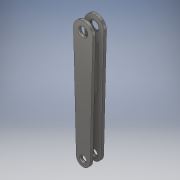
# Autodesk Inventor part: Upper Rocker Arm Spider Crab
Saved by Autodesk Inventor 2019 (Build 230136000, 136)
## iProperties
Created: 2019-08-25
Part Number: Upper Rocker Arm Spider Crab
Material: Steel, Mild
Document SubType Name: Modeling
Designer: DIBYOJYOTI
Density: 7.85 g/cm^3
Appearance: Semi-Polished
Mass: 46.5532 g
Surface Area: 51.0347 cm^2
Volume: 5.93034 cm^3
Author: DIBYOJYOTI
Autodesk Inventor part; units mm, degrees
ref_plane "YZ Plane" through (0, 0, 0) normal (1, 0, 0) x (0, 1, 0)
ref_plane "XZ Plane" through (0, 0, 0) normal (0, 1, 0) x (-1, 0, 0)
ref_plane "XY Plane" through (0, 0, 0) normal (0, 0, 1) x (1, 0, 0)
sketch "Sketch1" plane through (0, 0, 0) normal (0, 0, 1) x (1, 0, 0)
  circle A0 centre (0, 0) radius 2.05
  circle A1 centre (0, 80) radius 3.05
  arc A2 (6.9978, 79.8249) -> (-6.9978, 79.8249) centre (0, 80) ccw
  arc A3 (-5, 0) -> (5, 0) centre (0, 0) ccw
  line L0 (-5, 0) -> (-6.9978, 79.8249)
  line L1 (5, 0) -> (6.9978, 79.8249)
  dimension "d0" = 4.1
  dimension "d3" = 6.1
  dimension "d5" = 80
  dimension "d12" = 14
  dimension "d13" = 10
  constraints: 4 centre point, 4 end point, 4 point on circle, 3 coincident, 2 tangent
  measures "d0" diameter of A0
  measures "d3" diameter of A1
  measures "d5" distance of point (0, 0) A1.centre
  measures "d12" diameter of A2
  measures "d13" diameter of A3
extrude "Extrusion3" add sketch "Sketch1" along normal blind 10
fillet "Fillet2" radius 0.5 4 edges at (-3.05, 80, 10) (-3.05, 80, 0) (-2.05, 0, 10) (-2.05, 0, 0) curvature continuous yes
shell "Shell1" thickness 2 removed faces 4 at (4.486, 85.3736, 6.6667) at (5.6659, 26.6083, 3.3333) at (-6.3319, 53.2166, 3.3333) at (4.9838, -0.4023, 6.6667)
sketch "Sketch2" plane through (0, 80, 8) normal (0, 0, -1) x (-1, 0, 0)
  line L0 (0, -40) -> (-3, -40)
  line L1 (0, -10) -> (-3, -10)
  line L2 (-3, -40) -> (-3, -10)
  line L3 (0, -10) -> (3, -10)
  line L4 (0, -10) -> (3, -10) construction
  line L5 (3, -10) -> (3, -40)
  line L6 (3, -40) -> (0, -40)
  arc A0 (6.9978, -0.1751) -> (-6.9978, -0.1751) centre (0, 0) ccw projected
  point P0 (0, -80)
  dimension "d20" = 3
  dimension "d22" = 3
  dimension "d24" = 3
  dimension "d25" = 0
  dimension "d26" = 30
  dimension "d27" = 90
  dimension "d31" = 10
  constraints: 14 end point, 3 horizontal, 2 perpendicular, 1 collinear
  measures "d20" distance of L0.start L0.end
  measures "d22" distance of L1.start L1.end
  measures "d24" distance of L1.start L3.end
  measures "d25" distance between parallel lines of L3 L4
  measures "d26" distance of L3.end L5.end
  measures "d27" angle of L3 L5
  measures "d31" distance from line of A0.centre L3
extrude "Extrusion4" add sketch "Sketch2" along normal blind 6
delete faces "Delete Face1" heal yes whole lump no faces at (4.0369, 0.3259, 4) (2.0434, -0.165, 6.5)
delete faces "Delete Face2" heal yes whole lump no faces at (5.0336, 80.4064, 4) (3.0401, 79.7546, 6.5)
fillet "Fillet3" radius 0.5 4 edges at (-2.05, 0, 8) (-3.05, 80, 8) (-2.05, 0, 2) (-3.05, 80, 2) curvature continuous yes
body "Solid3"
